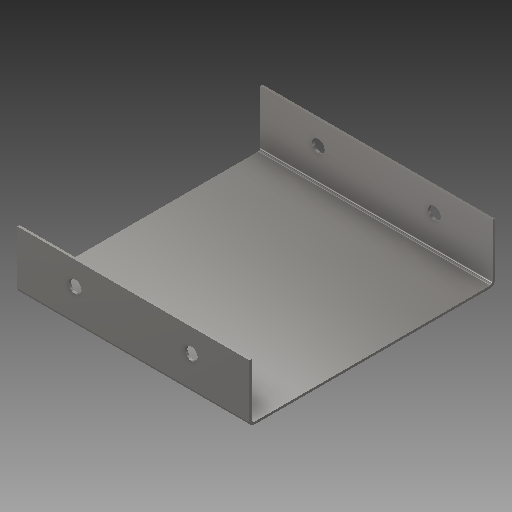
# Autodesk Inventor part: Sheet Metal Support
Saved by Autodesk Inventor 2019.4 (Build 234330000, 330)
## iProperties
Created: 2020-01-30
Part Number: Sheet Metal Support
Material: Steel, Alloy
Document SubType Name: Sheet Metal
Designer: Mark
Mass: 116.713 g
Surface Area: 308.059 cm^2
Volume: 15.0987 cm^3
Density: 7.73 g/cm^3
Sheet Metal Rule: Default_mm
Appearance: Semi-Polished
Author: Mark
Autodesk Inventor part; units mm, degrees
ref_plane "YZ Plane" through (0, 0, 0) normal (1, 0, 0) x (0, 1, 0)
ref_plane "XZ Plane" through (0, 0, 0) normal (0, 1, 0) x (-1, 0, 0)
ref_plane "XY Plane" through (0, 0, 0) normal (0, 0, 1) x (1, 0, 0)
sketch "Sketch1" plane through (0, 0, 0) normal (0, 1, 0) x (-1, 0, 0)
  line L0 (-50, 52.85) -> (50, 52.85)
  line L1 (50, 52.85) -> (50, -52.85)
  line L2 (50, -52.85) -> (-50, -52.85)
  line L3 (-50, -52.85) -> (-50, 52.85)
  line L4 (-50, 52.85) -> (50, -52.85) construction
  line L5 (50, 52.85) -> (-50, -52.85) construction
  point P0 (0, 0)
  dimension "d0" = 100
  dimension "d1" = 105.7
  measures "d0" distance of L1.end L2.end
  measures "d1" distance of L0.end L1.end
extrude "Plate1" add sketch "Sketch1" along normal blind 1
sketch "Sketch2" plane through (50, 0, 51.85) normal (0, 0, 1) x (1, 0, 0)
  line L0 (-100, 0) -> (0, 0)
  line L1 (0, 0) -> (0, 25)
  line L2 (0, 25) -> (-100, 25)
  line L3 (-100, 25) -> (-100, 0)
  constraints: 6 end point, 1 horizontal, 1 perpendicular, 1 vertical
edge flange "Flange1" height 25 angle 90 thickness 1 bend radius 1 thickness toward (0, 0, 1) relief straight relief width 1 relief depth 0.5 corner gap 1 corner form 0 edges at (0, 1, 52.85) (0, 1, -52.85) wall of the first edge with corners at (-50, 0, 51.85) (50, 0, 51.85) (50, 25, 51.85) (-50, 25, 51.85)
bend "Bend1"
corner "Corner1"
sketch "Sketch3" plane through (0, 1, 0) normal (0, 1, 0) x (1, 0, 0)
  circle A0 centre (25, -40.35) radius 2.75
  circle A1 centre (-25, -40.35) radius 2.75
  line L0 (50, 50.85) -> (50, -50.85) projected
  line L1 (-50, -52.85) -> (50, -52.85) projected
  point P0 (0, 0)
  dimension "d13" = 5.5
  dimension "d14" = 5.5
  dimension "d15" = 50
  dimension "d16" = 25
  dimension "d17" = 12.5
  dimension "d18" = 12.5
  constraints: 2 centre point
  measures "d13" diameter of A0
  measures "d14" diameter of A1
  measures "d15" distance of A0.centre A1.centre
  measures "d16" distance from line of L0 A0.centre
  measures "d17" distance from line of L1 A0.centre
  measures "d18" distance from line of L1 A1.centre
extrude "Extrusion1" cut sketch "Sketch3" against normal blind 10
sketch "Sketch4" plane through (-50, 25, 52.85) normal (0, 0, 1) x (1, 0, 0)
  circle A0 centre (25, -10) radius 2.75
  circle A1 centre (75, -10) radius 2.75
  line L0 (0, -23) -> (0, 0) projected
  line L1 (100, 0) -> (100, -23) projected
  line L2 (0, 0) -> (100, 0) projected
  point P0 (50, -25)
  dimension "d21" = 5.5
  dimension "d22" = 5.5
  dimension "d23" = 25
  dimension "d24" = 25
  dimension "d25" = 10
  dimension "d26" = 10
  constraints: 2 centre point
  measures "d21" diameter of A0
  measures "d22" diameter of A1
  measures "d23" distance from line of L0 A0.centre
  measures "d24" distance from line of L1 A1.centre
  measures "d25" distance from line of L2 A1.centre
  measures "d26" distance from line of L2 A0.centre
extrude "Extrusion2" cut sketch "Sketch4" against normal through all
equation "\"d2\" = Thickness"
equation "\"d3\" = BendReliefWidth"
equation "\"d4\" = BendReliefDepth"
equation "\"d5\" = MinimumRemnant"
equation "\"d6\" = TransitionRadius"
equation "\"d9\" = BendRadius"
equation "\"d10\" = CornerReliefSize"
equation "\"d11\" = GapSize"
equation "\"d12\" = JacobiRadiusSize"
equation "\"BendRadius\" = Thickness"
equation "\"BendReliefWidth\" = Thickness"
equation "\"BendReliefDepth\" = 0.5 * Thickness"
equation "\"CornerReliefSize\" = 4 * Thickness"
equation "\"MinimumRemnant\" = 2 * Thickness"
equation "\"TransitionRadius\" = BendRadius"
equation "\"JacobiRadiusSize\" = BendRadius"
equation "\"GapSize\" = Thickness"
equation "\"Thickness\" = 1"
body "Solid1"
